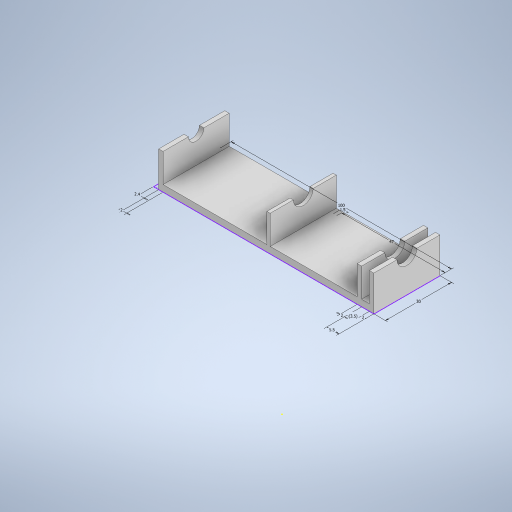
# Autodesk Inventor part: Hamilton 10 micL syringe holder
Saved by Autodesk Inventor 2023.2 (Build 272271000, 271)
## iProperties
Created: 2023-03-03
Part Number: Hamilton 10 micL syringe holder
Material: Generic
Document SubType Name: Modeling
Designer: dmargari
Density: 1 g/cm^3
Appearance: Default
Author: dmargari
## iProperties of the stored document Hamilton 10 micL syringe holder_3DPrint.ipt
Created: 2023-03-16
Part Number: Hamilton 10 micL syringe holder_3DPrint
Material: Generic
Document SubType Name: Modeling
Designer: dmargari
Density: 1 g/cm^3
Appearance: Default
Author: dmargari
Autodesk Inventor part; units mm, degrees
ref_plane "YZ Plane" through (0, 0, 0) normal (1, 0, 0) x (0, 1, 0)
ref_plane "XZ Plane" through (0, 0, 0) normal (0, 1, 0) x (-1, 0, 0)
ref_plane "XY Plane" through (0, 0, 0) normal (0, 0, 1) x (1, 0, 0)
sketch "Sketch1" plane through (0, 0, 0) normal (0, 1, 0) x (-1, 0, 0)
  line L0 (118.6192, -60.316) -> (18.6192, -60.316)
  line L1 (18.6192, -60.316) -> (18.6192, -90.316)
  line L2 (18.6192, -90.316) -> (118.6192, -90.316)
  line L3 (118.6192, -90.316) -> (118.6192, -60.316)
  line L4 (118.6192, -60.316) -> (18.6192, -90.316) construction
  line L5 (18.6192, -60.316) -> (118.6192, -90.316) construction
  line L6 (116.2192, -60.316) -> (116.2192, -90.316)
  line L7 (114.2192, -60.316) -> (114.2192, -90.316)
  line L8 (26.1192, -60.316) -> (26.1192, -90.316)
  line L9 (24.1192, -60.316) -> (24.1192, -90.316)
  line L10 (65.6192, -90.316) -> (65.6192, -60.316)
  line L11 (67.1192, -90.316) -> (67.1192, -60.316)
  line L12 (20.6192, -90.316) -> (20.6192, -60.316)
  point P0 (0, 0)
  point P1 (68.6192, -75.316)
  dimension "d0" = 100
  dimension "d1" = 30
  dimension "d2" = 2.4
  dimension "d3" = 2
  dimension "d4" = 5.5
  dimension "d5" = 2
  dimension "d24" = 47
  dimension "d25" = 1.5
  dimension "d28" = 2
  dimension "d29" = 3.5
  constraints: 22 end point, 8 vertical, 2 midpoint, 1 parallel, 20 other
  measures "d0" distance of L3.start L1.end
  measures "d1" distance of L1.end L1.start
  measures "d2" distance between parallel lines of L3 L6
  measures "d3" distance between parallel lines of L6 L7
  measures "d4" distance between parallel lines of L9 L1
  measures "d5" distance between parallel lines of L9 L8
  measures "d24" distance between parallel lines of L10 L1
  measures "d25" distance between parallel lines of L10 L11
  measures "d28" distance between parallel lines of L1 L12
  measures "d29" distance between parallel lines of L9 L12
extrude "Extrusion1" add sketch "Sketch1" along normal blind 3 contours L7 L2 L11 L0 | L10 L2 L8 L0 | L9 L2 L12 L0
extrude "Extrusion2" add sketch "Sketch1" along normal blind 16 contours L6 L2 L7 L0
extrude "Extrusion8" add sketch "Sketch1" along normal blind 16 contours L11 L2 L10 L0
extrude "Extrusion4" add sketch "Sketch1" along normal blind 16 contours L8 L2 L9 L0
extrude "Extrusion5" add sketch "Sketch1" along normal blind 3 contours L9 L2 L12 L0 | L12 L2 L1 L0
extrude "Extrusion9" add sketch "Sketch1" along normal blind 16 contours L12 L2 L1 L0
sketch "Sketch2" plane through (-18.6192, 16, -60.316) normal (1, 0, 0) x (0, 0, -1)
  line L0 (30, -13) -> (0, -13) construction
  line L1 (30, -13) -> (30, 0) construction
  line L2 (0, 0) -> (30, 0) construction
  line L3 (0, -13) -> (0, 0) construction
  line L4 (0, 0) -> (30, 0) construction
  line L5 (15, 0) -> (15, -13) construction
  line L6 (30, -13) -> (0, -13) construction
  circle A0 centre (15, 0) radius 4.5
  point P0 (-60.316, -16)
  dimension "d18" = 9
  constraints: 2 end point, 2 midpoint, 1 centre point, 1 coincident
  measures "d18" diameter of A0
extrude "Extrusion6" cut sketch "Sketch2" against normal up to surface (48.5 mm away)
sketch "Sketch3" plane through (-116.2192, 16, -90.316) normal (-1, 0, 0) x (0, 0, 1)
  line L0 (30, 0) -> (0, 0) projected
  circle A0 centre (15, 0) radius 3.5
  point P0 (90.316, -16)
  dimension "d19" = 7
  constraints: 1 centre point, 1 midpoint
  measures "d19" diameter of A0
extrude "Extrusion7" cut sketch "Sketch3" against normal up to surface (2 mm away)
body "Solid1"
